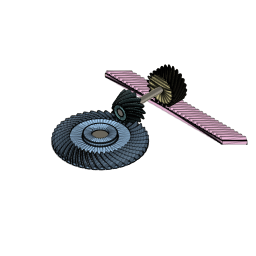
Gear train v1 (Autodesk Fusion 360 design; units mm, degrees)
Autodesk Fusion 360 part; units mm, degrees
other "Base Mesh Feature3"
other "Base Mesh Feature4"
sketch "Sketch1" plane through (0, 0, 0) normal (0, 1, 0) x (1, 0, 0)
  circle A0 centre (-15, -27) radius 4
extrude "Extrude1" add sketch "Sketch1" along normal blind 10 and the other way blind 75 makes body 1
other "Base Mesh Feature5"
sketch "Sketch2" plane through (0, -75, 0) normal (0, -1, 0) x (1, 0, 0)
  circle A0 centre (-15, 27) radius 4
  circle A1 centre (-15, 27) radius 5
extrude "Extrude2" add sketch "Sketch2" along normal blind 0 and the other way blind 19.75 bodies 1
other "Base Mesh Feature7"
other "Modify1"
other "Modify2"
sketch "Sketch3" plane through (0, 0, 0) normal (0, 0, 1) x (1, 0, 0)
  circle A0 centre (-12.1217, -110.1546) radius 10
  dimension "d9" = 20
  measures "d9" diameter of A0
extrude "Extrude3" add sketch "Sketch3" along normal blind 15 and the other way blind 20 separate body makes body 2
